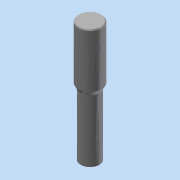
# Autodesk Inventor part: reservoir
Saved by Autodesk Inventor 2017 (Build 210142000, 142)
## iProperties
Created: 2018-04-14
Part Number: reservoir
Material: S235JR (E24-2)
Document SubType Name: Modeling
Designer: RozierB
Density: 7.85 g/cm^3
Appearance: Acier
Author: RozierB
Autodesk Inventor part; units mm, degrees
ref_plane "YZ Plane" through (0, 0, 0) normal (1, 0, 0) x (0, 1, 0)
ref_plane "XZ Plane" through (0, 0, 0) normal (0, 1, 0) x (-1, 0, 0)
ref_plane "XY Plane" through (0, 0, 0) normal (0, 0, 1) x (1, 0, 0)
sketch "Esquisse4" plane through (0, 0, 0) normal (1, 0, 0) x (0, 1, 0)
  line L0 (26, -2) -> (26, -121)
  line L1 (24, 0) -> (0, 0)
  line L2 (0, 0) -> (0, -6)
  line L3 (0, -6) -> (18, -6)
  line L4 (20, -106) -> (10, -126)
  line L5 (20, -106) -> (20, -8)
  line L6 (20, -8) -> (18, -6)
  line L7 (24, 0) -> (26, -2)
  line L8 (10, -126) -> (10, -130.5)
  line L9 (10, -130.5) -> (10.5, -131)
  line L10 (10.5, -131) -> (12.6076, -131)
  arc A0 (12.6076, -131) -> (12.8342, -130.6443) centre (12.6076, -130.75) ccw
  line L11 (12.8342, -130.6443) -> (12.1462, -129.169)
  arc A1 (12.5087, -128.6) -> (12.1462, -129.169) centre (12.5087, -129) ccw
  line L12 (12.5087, -128.6) -> (15.8913, -128.6)
  arc A2 (16.2538, -129.169) -> (15.8913, -128.6) centre (15.8913, -129) ccw
  line L13 (16.2538, -129.169) -> (15.5658, -130.6443)
  arc A3 (15.5658, -130.6443) -> (15.7924, -131) centre (15.7924, -130.75) ccw
  line L14 (15.7924, -131) -> (17.5, -131)
  line L15 (15.5658, -130.6443) -> (15.4, -131) construction
  line L16 (15.4, -131) -> (15.7924, -131) construction
  line L17 (12.8342, -130.6443) -> (13, -131) construction
  line L18 (13, -131) -> (12.6076, -131) construction
  line L19 (17.5, -131) -> (18.5, -132)
  line L20 (26, -121) -> (21, -131)
  line L21 (21, -271) -> (21, -131)
  line L22 (18, -271) -> (21, -271)
  line L23 (0, -325.2) -> (0, 54.2) projected
  line L24 (18.5, -132) -> (18.5, -138.5)
  line L25 (18.5, -138.5) -> (18, -139)
  line L26 (18, -139) -> (18, -271)
  dimension "d11" = 2
  dimension "d12" = 6
  dimension "d13" = 6
  dimension "d14" = 2
  dimension "d15" = 2
  dimension "d16" = 2
  dimension "d17" = 65
  dimension "d18" = 0.25
  dimension "d19" = 0.4
  dimension "d20" = 65
  dimension "d21" = 2.4
  dimension "d22" = 2.4
  dimension "d23" = 0.5
  dimension "d24" = 0.5
  dimension "d25" = 3
  dimension "d26" = 20
  dimension "d27" = 20
  dimension "d28" = 100
  dimension "d29" = 10
  dimension "d30" = 5
  dimension "d35" = 1
  dimension "d37" = 1
  dimension "d46" = 140
  dimension "d64" = 18
  dimension "d65" = 0.5
  dimension "d68" = 0.5
  dimension "d72" = 8
  dimension "d75" = 3
  constraints: 52 end point, 8 point on circle, 8 tangent, 5 collinear, 5 horizontal, 4 centre point, 4 vertical, 3 perpendicular, 2 equal radius, 1 coincident, 1 horizontal alignment, 1 parallel
  measures "d11" horizontal distance of L1.start L0.start
  measures "d12" distance between parallel lines of L3 L1
  measures "d13" distance between parallel lines of L0 L5
  measures "d14" horizontal distance of L1.start L0.start
  measures "d15" horizontal distance of L5.end L3.end
  measures "d16" horizontal distance of L5.end L3.end
  measures "d17" angle of L11 L10
  measures "d18" radius of A0
  measures "d19" radius of A1
  measures "d20" angle of L13 L14
  measures "d21" distance of L17.end L15.end
  measures "d22" distance from line of L12 L15.end
  measures "d23" horizontal distance of L8.end L9.end
  measures "d24" horizontal distance of L8.end L9.end
  measures "d25" distance from line of L8 L17.end
  measures "d26" distance between parallel lines of L2 L5
  measures "d27" vertical distance of L4.start L4.end
  measures "d28" distance from line of L4.start L3
  measures "d29" distance between parallel lines of L2 L8
  measures "d30" vertical distance of L9.end L4.end
  measures "d35" horizontal distance of L14.end L19.end
  measures "d37" horizontal distance of L14.end L19.end
  measures "d46" distance from line of L22.start L14
  measures "d64" distance between parallel lines of L23 L26
  measures "d65" distance between parallel lines of L24 L26
  measures "d68" horizontal distance of L24.end L25.end
  measures "d72" distance from line of L14 L25.end
  measures "d75" distance between parallel lines of L21 L26
revolve "Révolution1" add sketch "Esquisse4" angle 360 about axis through (0, 0, -10) along (0, 0, 1)
sketch "Esquisse5" plane through (0, 0, 0) normal (1, 0, 0) x (0, 1, 0)
  line L0 (-26, -2) -> (-24, 0) projected
  line L1 (-24, 0) -> (24, 0) projected
  line L2 (24, 0) -> (26, -2) projected
  line L3 (26, -2) -> (26, -121) projected
  line L4 (26, -121) -> (21, -131) projected
  line L5 (21, -131) -> (21, -271) projected
  line L6 (21, -271) -> (18, -271) projected
  line L7 (18.5, -132) -> (17.5, -131) projected
  line L8 (17.5, -131) -> (15.7924, -131) projected
  arc A0 (15.5658, -130.6443) -> (15.7924, -131) centre (15.7924, -130.75) ccw projected
  line L9 (15.5658, -130.6443) -> (16.2538, -129.169) projected
  arc A1 (16.2538, -129.169) -> (15.8913, -128.6) centre (15.8913, -129) ccw projected
  line L10 (15.8913, -128.6) -> (12.5087, -128.6) projected
  arc A2 (12.5087, -128.6) -> (12.1462, -129.169) centre (12.5087, -129) ccw projected
  line L11 (12.1462, -129.169) -> (12.8342, -130.6443) projected
  arc A3 (12.6076, -131) -> (12.8342, -130.6443) centre (12.6076, -130.75) ccw projected
  line L12 (12.6076, -131) -> (10.5, -131) projected
  line L13 (10.5, -131) -> (10, -130.5) projected
  line L14 (10, -130.5) -> (10, -126) projected
  line L15 (10, -126) -> (20, -106) projected
  line L16 (20, -106) -> (20, -8) projected
  line L17 (20, -8) -> (18, -6) projected
  line L18 (18, -6) -> (-18, -6) projected
  line L19 (-18, -6) -> (-20, -8) projected
  line L20 (-20, -8) -> (-20, -106) projected
  line L21 (-20, -106) -> (-10, -126) projected
  line L22 (-10, -126) -> (-10, -130.5) projected
  line L23 (-10, -130.5) -> (-10.5, -131) projected
  line L24 (-10.5, -131) -> (-12.6076, -131) projected
  arc A4 (-12.8342, -130.6443) -> (-12.6076, -131) centre (-12.6076, -130.75) ccw projected
  line L25 (-12.8342, -130.6443) -> (-12.1462, -129.169) projected
  arc A5 (-12.1462, -129.169) -> (-12.5087, -128.6) centre (-12.5087, -129) ccw projected
  line L26 (-12.5087, -128.6) -> (-15.8913, -128.6) projected
  arc A6 (-15.8913, -128.6) -> (-16.2538, -129.169) centre (-15.8913, -129) ccw projected
  line L27 (-16.2538, -129.169) -> (-15.5658, -130.6443) projected
  arc A7 (-15.7924, -131) -> (-15.5658, -130.6443) centre (-15.7924, -130.75) ccw projected
  line L28 (-15.7924, -131) -> (-17.5, -131) projected
  line L29 (-17.5, -131) -> (-18.5, -132) projected
  line L30 (-18, -271) -> (-21, -271) projected
  line L31 (-21, -271) -> (-21, -131) projected
  line L32 (-21, -131) -> (-26, -121) projected
  line L33 (-26, -121) -> (-26, -2) projected
  line L34 (18, -136) -> (0, -136)
  line L35 (0, -189) -> (10.75, -189)
  line L36 (10.75, -189) -> (11, -188.75)
  line L37 (11, -188.75) -> (11, -139.5)
  line L38 (11, -139.5) -> (11.5, -139)
  line L39 (11.5, -139) -> (18, -139)
  line L40 (18, -139) -> (18.5, -138.5)
  line L41 (18.5, -138.5) -> (18.5, -136.5)
  line L42 (18.5, -136.5) -> (18, -136)
  line L43 (0, -277.2) -> (0, 46.2) projected
  line L44 (-18, -136) -> (0, -136)
  line L45 (0, -189) -> (-10.75, -189)
  line L46 (-10.75, -189) -> (-11, -188.75)
  line L47 (-11, -188.75) -> (-11, -139.5)
  line L48 (-11, -139.5) -> (-11.5, -139)
  line L49 (-11.5, -139) -> (-18, -139)
  line L50 (-18, -139) -> (-18.5, -138.5)
  line L51 (-18.5, -138.5) -> (-18.5, -136.5)
  line L52 (-18.5, -136.5) -> (-18, -136)
  line L53 (18, -271) -> (18, -139) projected
  line L54 (18, -139) -> (18.5, -138.5) projected
  line L55 (18.5, -138.5) -> (18.5, -132) projected
  line L56 (-18.5, -132) -> (-18.5, -138.5) projected
  line L57 (-18.5, -138.5) -> (-18, -139) projected
  line L58 (-18, -139) -> (-18, -271) projected
  point P0 (0, 0)
  dimension "d49" = 3
  dimension "d50" = 5
  dimension "d51" = 0.5
  dimension "d52" = 0.5
  dimension "d53" = 0.5
  dimension "d54" = 0.5
  dimension "d55" = 11
  dimension "d56" = 18.5
  dimension "d57" = 0.5
  dimension "d58" = 0.5
  dimension "d59" = 0.25
  dimension "d60" = 0.25
  dimension "d61" = 50
  constraints: 36 end point, 8 symmetric about line, 2 horizontal, 2 perpendicular, 2 point on line
  measures "d49" distance between parallel lines of L39 L34
  measures "d50" distance between parallel lines of L34 L12
  measures "d51" horizontal distance of L41.end L34.start
  measures "d52" horizontal distance of L41.end L34.start
  measures "d53" horizontal distance of L39.end L40.end
  measures "d54" horizontal distance of L39.end L40.end
  measures "d55" distance between parallel lines of L37 L43
  measures "d56" distance between parallel lines of L41 L43
  measures "d57" horizontal distance of L37.end L38.end
  measures "d58" horizontal distance of L37.end L38.end
  measures "d59" horizontal distance of L35.end L36.end
  measures "d60" horizontal distance of L35.end L36.end
  measures "d61" distance between parallel lines of L39 L35
extrude "Extrusion4" cut sketch "Esquisse5" against normal up to surface contours L34 L42 L41 L40 L39 L38 L37 L36 L35 L43 | L43 L45 L46 L47 L48 L49 L50 L51 L52 L44
equation "\"d11\" = d14"
equation "\"d16\" = d15"
equation "\"d20\" = d17"
equation "\"d24\" = d23"
